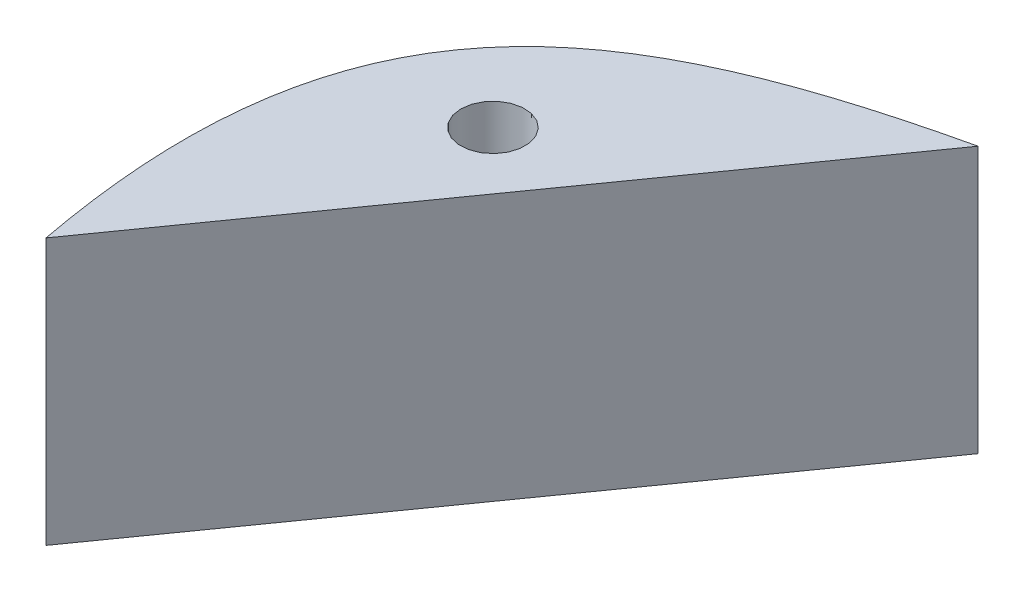
# Autodesk Inventor part: Rear_Strut_pivot_support
Saved by Autodesk Inventor 2016 (Build 200138000, 138)
## iProperties
Created: 2015-08-10
Part Number: Rear_Strut_pivot_support
Material: Generic
Document SubType Name: Modeling
Designer: Yann
Density: 1 g/cm^3
Appearance: Default
Author: Yann
Autodesk Inventor part; units mm, degrees
ref_plane "YZ Plane" through (0, 0, 0) normal (1, 0, 0) x (0, 1, 0)
ref_plane "XZ Plane" through (0, 0, 0) normal (0, 1, 0) x (-1, 0, 0)
ref_plane "XY Plane" through (0, 0, 0) normal (0, 0, 1) x (1, 0, 0)
sketch "Sketch1" plane through (0, 0, 0) normal (0, 1, 0) x (-1, 0, 0)
  spline S0 degree 4 poles (-828.8768, -38.004) (-800.9087, -82.7506) (-658.226, -367.9632) (-748.0807, -311.2325) (-933.0769, -357.0897) knots 1 1 1 1 1 2 2 2 2 2 projected
  line L0 (-747.2163, -232.4548) -> (-819.4295, -334.3508) construction
  spline S1 degree 1 poles (-747.2163, -232.4548) (-819.4295, -334.3508) knots 1 1 2 2
  circle A0 centre (-771.0847, -292.076) radius 6
  line L1 (-783.3229, -283.4028) -> (-771.0847, -292.076) construction
  point P0 (0, 0)
  dimension "d0" = 12
  dimension "d1" = 15
  constraints: 2 coincident, 2 end point, 1 centre point, 1 midpoint, 1 perpendicular, 1 symmetric about line, 8 other
  measures "d0" diameter of A0
  measures "d1" distance of L1.start L1.end
extrude "Extrusion1" add sketch "Sketch1" along normal mid plane 49.75
body "Solid1"
